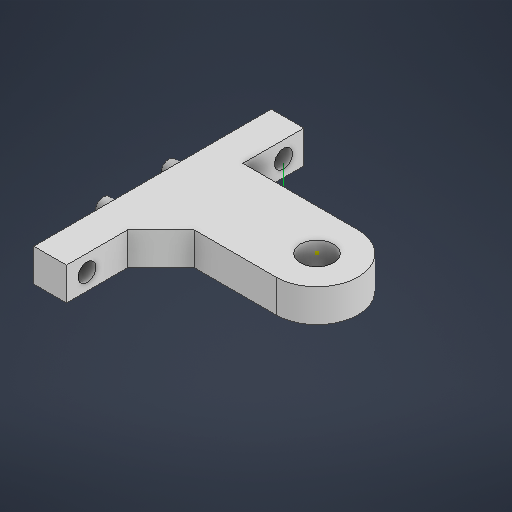
# Autodesk Inventor part: Launcher_support
Saved by Autodesk Inventor 2026.1 (Build 301233020, 233B)
## iProperties
Created: 2025-10-31
Part Number: Launcher_support
Material: Generic
Document SubType Name: Modeling
Designer: Asus
Density: 1 g/cm^3
Appearance: Default
Author: Asus
Autodesk Inventor part; units mm, degrees
ref_plane "YZ Plane" through (0, 0, 0) normal (1, 0, 0) x (0, 1, 0)
ref_plane "XZ Plane" through (0, 0, 0) normal (0, 1, 0) x (-1, 0, 0)
ref_plane "XY Plane" through (0, 0, 0) normal (0, 0, 1) x (1, 0, 0)
sketch "Sketch1" plane through (0, 0, 0) normal (0, 1, 0) x (-1, 0, 0)
  circle A0 centre (0, 0) radius 4.025
  line L0 (0, 0) -> (36.11, 0) construction
  line L1 (0, -10) -> (36.11, -10)
  line L2 (36.11, 10) -> (0, 10)
  arc A1 (0, 10) -> (0, -10) centre (0, 0) ccw
  line L3 (36.11, 10) -> (36.11, -10)
  point P0 (18.055, 0)
  dimension "d0" = 8.05
  dimension "d1" = 36.11
  constraints: 10 end point, 2 centre point, 2 point on circle, 2 tangent, 1 coincident, 1 horizontal, 1 midpoint, 1 parallel, 1 vertical
  measures "d0" diameter of A0
  measures "d1" distance of L0.start L0.end
extrude "Extrusion1" add sketch "Sketch1" along normal blind 8
sketch "Sketch2" plane through (-36.11, 0, 10) normal (0, 0, 1) x (1, 0, 0)
  line L0 (0, 0) -> (0, 8) projected
  line L1 (36.11, 0) -> (0, 0) projected
  line L2 (0, 8) -> (8, 8)
  line L3 (8, 8) -> (8, 0)
  line L4 (8, 0) -> (0, 0)
  line L5 (0, 0) -> (0, 8)
  dimension "d5" = 8
  constraints: 8 end point, 2 parallel, 1 horizontal, 1 perpendicular, 1 point on line
  measures "d5" distance of L3.end L4.end
extrude "Extrusion2" add sketch "Sketch2" along normal blind 23.06
sketch "Sketch3" plane through (-28.11, 0, 10) normal (1, 0, 0) x (0, 0, -1)
  circle A0 centre (-18.06, 4) radius 2.2
  line L0 (-23.06, 0) -> (-23.06, 8) projected
  point P0 (10, 0)
  point P1 (-23.06, 4)
  dimension "d8" = 4.4
  dimension "d9" = 5
  constraints: 1 centre point, 1 midpoint
  measures "d8" diameter of A0
  measures "d9" distance of point (-23.06, 4) A0.centre
extrude "Extrusion3" cut sketch "Sketch3" against normal blind 23.06
sketch "Sketch4" plane through (0, 0, -10) normal (0, 0, -1) x (-1, 0, 0)
  line L0 (36.11, 0) -> (36.11, 8) projected
  line L1 (28.11, 0) -> (28.11, 8) projected
  line L2 (36.11, 8) -> (28.11, 8)
  line L3 (28.11, 8) -> (28.11, 0)
  line L4 (28.11, 0) -> (36.11, 0)
  line L5 (36.11, 0) -> (36.11, 8)
  point P0 (0, 0)
  constraints: 8 end point, 2 parallel, 1 horizontal, 1 perpendicular
extrude "Extrusion4" add sketch "Sketch4" along normal blind 14.94
sketch "Sketch6" plane through (-36.11, 0, 33.06) normal (-1, 0, 0) x (0, 0, 1)
  circle A0 centre (-21, 4) radius 1.95
  circle A1 centre (-5, 4) radius 2.2 projected
  circle A2 centre (-37, 4) radius 1.95
  circle A3 centre (-53, 4) radius 2.2
  point P0 (-33.06, 0)
  dimension "d18" = 3.9
  dimension "d19" = 16
  dimension "d20" = 3.9
  dimension "d21" = 16
  dimension "d22" = 4.4
  dimension "d23" = 16
  constraints: 3 centre point
  measures "d18" diameter of A0
  measures "d19" distance of A1.centre A0.centre
  measures "d20" diameter of A2
  measures "d21" distance of A0.centre A2.centre
  measures "d22" diameter of A3
  measures "d23" distance of A2.centre A3.centre
extrude "Extrusion6" add sketch "Sketch6" along normal blind 4 contours A0 | A2
extrude "Extrusion7" cut sketch "Sketch6" against normal blind 13 contours A3
sketch "Sketch7" plane through (0, 8, 0) normal (0, 1, 0) x (1, 0, 0)
  point P0 (0, 0)
sketch "Sketch8" plane through (0, 8, 0) normal (0, 1, 0) x (1, 0, 0)
  line L0 (-28.11, -10) -> (-28.11, -33.06) construction
  line L1 (-28.11, -28.0914) -> (-28.11, -18.1514)
  line L2 (-28.11, -18.1514) -> (-19.9586, -10)
  line L3 (-28.11, -10) -> (0, -10) projected
  line L4 (-28.11, -18.1514) -> (-16.5822, -18.1514) construction
  line L5 (-19.9586, -10) -> (-28.11, -10)
  line L6 (-28.11, -10) -> (-28.11, -18.1514)
  point P0 (0, 0)
  dimension "d31" = 9.94
  dimension "d32" = 45
  constraints: 10 end point, 3 point on line, 2 collinear, 1 equal length, 1 horizontal
  measures "d31" distance of L1.start L1.end
  measures "d32" angle of L4 L2
extrude "Extrusion8" add sketch "Sketch8" against normal blind 8
body "Solid1"
